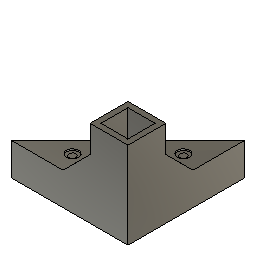
Rear Corner Bracket (Autodesk Fusion 360 design; units mm, degrees)
Autodesk Fusion 360 part; units mm, degrees
sketch "Sketch1" plane through (0, 0, 0) normal (0, 0, 1) x (1, 0, 0)
  line L0 (44, 14) -> (-44, 14)
  line L1 (-44, 14) -> (-44, -14)
  line L2 (-44, -14) -> (44, -14)
  line L3 (44, -14) -> (44, 14)
  line L4 (44, 14) -> (-44, -14) construction
  line L5 (-44, 14) -> (44, -14) construction
  dimension "d1" = 88
  dimension "d2" = 28
  constraint perpendicular L0 L1
  constraint parallel L0 L2
  constraint parallel L1 L3
  constraint horizontal L0
  constraint coincident L4 origin
  constraint coincident L5 origin
  measures "d1" distance of L1.end L2.end
  measures "d2" distance of L0.end L1.end
extrude "Extrude1" add sketch "Sketch1" along normal blind 24
sketch "Sketch2" plane through (0, 14, 0) normal (0, 1, 0) x (-1, 0, 0)
  line L0 (-44, 0) -> (44, 0)
  line L1 (44, 0) -> (44, 24)
  line L2 (44, 24) -> (-44, 24)
  line L3 (-44, 24) -> (-44, 0)
  line L4 (-44, 24) -> (-16, 24)
  line L5 (-16, 24) -> (-16, 0)
  line L6 (-16, 0) -> (-44, 0)
  line L7 (-44, 0) -> (-44, 24)
  dimension "d5" = 24
  dimension "d6" = 28
  constraint horizontal L4
  constraint vertical L5
  constraint horizontal L6
  constraint vertical L7
  constraint coincident L2.end L3.start
  measures "d5" distance of L2.end L0.start
  measures "d6" distance of L2.end L4.end
extrude "Extrude2" add sketch "Sketch2" along normal blind 60 contours L0 L2 L3 L4 L5 L6 L7
sketch "Sketch3" plane through (0, 0, 0) normal (0, 0, -1) x (1, 0, 0)
  line L0 (44, -74) -> (44, 14)
  line L1 (44, 14) -> (-44, 14)
  line L2 (-44, 14) -> (-44, -14)
  line L3 (-44, -14) -> (16, -14)
  line L4 (16, -14) -> (16, -74)
  line L5 (16, -74) -> (44, -74)
  line L6 (-44, 10) -> (44, 10) construction
  line L7 (-44, -10) -> (44, -10) construction
  line L8 (20, -74) -> (20, 14) construction
  line L9 (40, -74) -> (40, 14) construction
  line L10 (-44, 10) -> (40, 10)
  line L11 (40, 10) -> (40, -10)
  line L12 (40, -10) -> (-44, -10)
  line L13 (-44, -10) -> (-44, 10)
  line L14 (20, 10) -> (40, 10)
  line L15 (40, 10) -> (40, -74)
  line L16 (40, -74) -> (20, -74)
  line L17 (20, -74) -> (20, 10)
  dimension "d9" = 4
  dimension "d10" = 4
  dimension "d11" = 4
  dimension "d12" = 4
  constraint coincident L2 L6.start
  constraint coincident L0 L6.end
  constraint perpendicular L0 L6
  constraint coincident L2 L7.start
  constraint coincident L0 L7.end
  constraint perpendicular L0 L7
  constraint coincident L5 L8.start
  constraint coincident L1 L8.end
  constraint perpendicular L1 L8
  constraint coincident L5 L9.start
  constraint coincident L1 L9.end
  constraint perpendicular L1 L9
  constraint horizontal L10
  constraint vertical L11
  constraint horizontal L12
  constraint vertical L13
  constraint coincident L7 L11.end
  constraint coincident L9 L11.end
  constraint horizontal L14
  constraint vertical L15
  constraint horizontal L16
  constraint vertical L17
  constraint coincident L8 L14.start
  constraint coincident L10 L14.start
  measures "d9" distance of L0 L9
  measures "d10" distance of L4 L8
  measures "d11" distance of L3 L7
  measures "d12" distance of L1 L6
extrude "Extrude3" cut sketch "Sketch3" against normal blind 20 contours L5 L12 L15 L16 L17 | L10 L11 L12 L14 L15 L17 | L2 L10 L12 L13 L17
sketch "Sketch4" plane through (0, 0, 24) normal (0, 0, 1) x (-1, 0, 0)
  line L0 (-44, 14) -> (-44, -74)
  line L1 (-44, -74) -> (-16, -74)
  line L2 (-16, -74) -> (-16, -14)
  line L3 (-16, -14) -> (44, -14)
  line L4 (44, -14) -> (44, 14)
  line L5 (44, 14) -> (-44, 14)
  line L6 (14, -14) -> (-16, -44)
  constraint midpoint L3 L6.start
  constraint midpoint L2 L6.end
extrude "Extrude4" add sketch "Sketch4" against normal blind 4 contours L2 L3 L6
sketch "Sketch5" plane through (0, 0, 0) normal (0, 0, -1) x (1, 0, 0)
  line L0 (20, -10) -> (-44, -10)
  line L1 (-44, -10) -> (-44, -14)
  line L2 (-44, -14) -> (16, -14)
  line L3 (16, -14) -> (16, -74)
  line L4 (16, -74) -> (20, -74)
  line L5 (20, -74) -> (20, -10)
  line L6 (-14, -14) -> (16, -44)
  constraint midpoint L2 L6.start
  constraint midpoint L3 L6.end
extrude "Extrude5" add sketch "Sketch5" against normal blind 4 contours L2 L3 L6
sketch "Sketch6" plane through (0, 14, 0) normal (0, 1, 0) x (-1, 0, 0)
  line L0 (-16, 4) -> (14, 4)
  line L1 (14, 4) -> (14, 0)
  line L2 (14, 0) -> (44, 0)
  line L3 (44, 0) -> (44, 24)
  line L4 (44, 24) -> (14, 24)
  line L5 (14, 24) -> (14, 20)
  line L6 (14, 20) -> (-16, 20)
  line L7 (-16, 20) -> (-16, 4)
  line L8 (-6, 20) -> (-6, 4) construction
  line L9 (-16, 10) -> (44, 10) construction
  line L10 (14, 24) -> (-16, 24) construction
  circle A0 centre (-6, 10) radius 2.5
  circle A1 centre (-6, 10) radius 4.5
  dimension "d19" = 10
  dimension "d69" = 10
  dimension "d70" = 5
  dimension "d71" = 9
  constraint coincident L6 L8.start
  constraint coincident L0 L8.end
  constraint perpendicular L0 L8
  constraint coincident L7 L9.start
  constraint coincident L3 L9.end
  constraint perpendicular L3 L9
  constraint coincident L9 A0.centre
  constraint coincident L8 A0.centre
  constraint concentric A0 A1
  measures "d19" distance of L7 L8
  measures "d69" distance of L2 L9
  measures "d70" diameter of A0
  measures "d71" diameter of A1
extrude "Extrude36" cut sketch "Sketch6" against normal blind 1 contours A0 | A1
extrude "Extrude19" cut sketch "Sketch6" against normal blind 2.8 from surface at -1 contours A0
sketch "Sketch7" plane through (16, 0, 0) normal (-1, 0, 0) x (0, -1, 0)
  line L0 (-44, 0) -> (-44, 4)
  line L1 (-44, 4) -> (-14, 4)
  line L2 (-14, 4) -> (-14, 20)
  line L3 (-14, 20) -> (-44, 20)
  line L4 (-44, 20) -> (-44, 24)
  line L5 (-44, 24) -> (-74, 24)
  line L6 (-74, 24) -> (-74, 0)
  line L7 (-74, 0) -> (-44, 0)
  line L8 (-24, 20) -> (-24, 4) construction
  line L9 (-14, 20) -> (-14, 4) construction
  line L10 (-14, 10) -> (-74, 10) construction
  line L11 (-14, 24) -> (-44, 24) construction
  circle A0 centre (-24, 10) radius 2.5
  circle A1 centre (-24, 10) radius 4.5
  dimension "d26" = 10
  dimension "d62" = 5
  dimension "d63" = 9
  dimension "d76" = 10
  constraint coincident L3 L8.start
  constraint coincident L1 L8.end
  constraint perpendicular L1 L8
  constraint coincident L2 L10.start
  constraint coincident L6 L10.end
  constraint perpendicular L6 L10
  constraint coincident L8 A0.centre
  constraint coincident L10 A0.centre
  constraint concentric A0 A1
  measures "d26" distance of L8 L9
  measures "d62" diameter of A0
  measures "d63" diameter of A1
  measures "d76" distance of L7 L10
extrude "Extrude35" cut sketch "Sketch7" against normal blind 1 contours A0 | A1
extrude "Extrude17" cut sketch "Sketch7" against normal blind 2.8 from surface at -1 contours A0
sketch "Sketch8" plane through (0, 0, 24) normal (0, 0, 1) x (-1, 0, 0)
  line L0 (-44, 14) -> (-44, -74)
  line L1 (-44, -74) -> (-16, -74)
  line L2 (-16, -74) -> (-16, -44)
  line L3 (-16, -44) -> (14, -14)
  line L4 (14, -14) -> (44, -14)
  line L5 (44, -14) -> (44, 14)
  line L6 (44, 14) -> (-44, 14)
  line L7 (14, -14) -> (42, 14)
  line L8 (-16, -44) -> (-44, -72)
  constraint coincident L3.end L4.start
  constraint coincident L6 L7.end
  constraint parallel L3 L7
  constraint coincident L2.end L3.start
  constraint coincident L0 L8.end
  constraint parallel L3 L8
extrude "Extrude10" cut sketch "Sketch8" against normal blind 24 contours L0 L1 L2 L8 | L4 L5 L6 L7
sketch "Sketch11" plane through (0, 0, 24) normal (0, 0, 1) x (-1, 0, 0)
  line L0 (-44, -72) -> (42, 14)
  line L1 (42, 14) -> (-44, 14)
  line L2 (-44, 14) -> (-44, -72)
  line L3 (11, 14) -> (11, -17) construction
  line L4 (-44, -41) -> (-13, -41) construction
  line L5 (-30, 14) -> (-30, -58) construction
  line L6 (-44, 0) -> (28, 0) construction
  circle A0 centre (-30, -41) radius 2.5
  circle A1 centre (-30, -41) radius 4.5
  circle A2 centre (11, 0) radius 2.5
  circle A3 centre (11, 0) radius 4.5
  dimension "d49" = 55
  dimension "d50" = 55
  dimension "d51" = 14
  dimension "d52" = 14
  dimension "d53" = 5
  dimension "d54" = 9
  dimension "d55" = 5
  dimension "d56" = 9
  constraint coincident L1 L3.start
  constraint coincident L0 L3.end
  constraint perpendicular L1 L3
  constraint coincident L2 L4.start
  constraint coincident L0 L4.end
  constraint perpendicular L2 L4
  constraint coincident L1 L5.start
  constraint coincident L0 L5.end
  constraint perpendicular L1 L5
  constraint coincident L2 L6.start
  constraint coincident L0 L6.end
  constraint perpendicular L2 L6
  constraint coincident L4 A0.centre
  constraint coincident L5 A0.centre
  constraint concentric A0 A1
  constraint coincident L3 A2.centre
  constraint coincident L6 A2.centre
  constraint concentric A2 A3
  measures "d49" distance of L2 L3
  measures "d50" distance of L1 L4
  measures "d51" distance of L1 L6
  measures "d52" distance of L2 L5
  measures "d53" diameter of A0
  measures "d54" diameter of A1
  measures "d55" diameter of A2
  measures "d56" diameter of A3
extrude "Extrude16" cut sketch "Sketch11" against normal blind 1 contours A1 | A3
extrude "Extrude15" cut sketch "Sketch11" against normal blind 4 contours A0 | A2
sketch "Sketch13" plane through (0, 0, 23) normal (0, 0, 1) x (-1, 0, 0)
  circle A0 centre (-30, -41) radius 2.5
  circle A1 centre (-30, -41) radius 4.5
  circle A2 centre (-30, -41) radius 2.5
  circle A3 centre (-30, -41) radius 2.5
  constraint concentric A0 A2
  constraint concentric A2 A3
extrude "Extrude21" add sketch "Sketch11" against normal blind 0.2 from surface at -1 contours A0
sketch "Sketch14" plane through (0, 0, 23) normal (0, 0, 1) x (-1, 0, 0)
  circle A0 centre (11, 0) radius 2.5
  circle A1 centre (11, 0) radius 4.5
extrude "Extrude22" add sketch "Sketch11" along normal blind 0.2 from surface at -1.2 contours A2
sketch "Sketch16" plane through (0, 0, 24) normal (0, 0, 1) x (-1, 0, 0)
  circle A0 centre (11, 0) radius 4.5
  circle A1 centre (-30, -41) radius 4.5
  line L0 (-44, -72) -> (42, 14)
  line L1 (42, 14) -> (-44, 14)
  line L2 (-44, 14) -> (-44, -72)
  line L3 (-44, 14) -> (-16, 14)
  line L4 (-16, 14) -> (-16, -14)
  line L5 (-16, -14) -> (-44, -14)
  line L6 (-44, -14) -> (-44, 14)
  dimension "d83" = 28
  dimension "d84" = 28
  constraint horizontal L3
  constraint vertical L4
  constraint horizontal L5
  constraint vertical L6
  constraint coincident L1.end L2.start
  measures "d83" distance of L1.end L3.end
  measures "d84" distance of L1.end L5.end
extrude "Extrude23" add sketch "Sketch16" along normal blind 40 contours L1 L2 L3 L4 L5 L6
sketch "Sketch17" plane through (0, 0, 64) normal (0, 0, 1) x (-1, 0, 0)
  line L0 (-44, -14) -> (-16, -14)
  line L1 (-16, -14) -> (-16, 14)
  line L2 (-16, 14) -> (-44, 14)
  line L3 (-44, 14) -> (-44, -14)
  line L4 (-16, 0) -> (-18.5204, 0) construction
  line L5 (-18.5204, 0) -> (-44, 0) construction
  line L6 (-30, -14) -> (-30, 14) construction
  line L7 (-40, 10) -> (-20, 10)
  line L8 (-20, 10) -> (-20, -10)
  line L9 (-20, -10) -> (-40, -10)
  line L10 (-40, -10) -> (-40, 10)
  line L11 (-40, 10) -> (-20, -10) construction
  line L12 (-20, 10) -> (-40, -10) construction
  point P0 (-30, 0)
  dimension "d87" = 20
  dimension "d88" = 20
  constraint midpoint L1 L4.start
  constraint perpendicular L1 L4
  constraint midpoint L3 L5.end
  constraint perpendicular L3 L5
  constraint midpoint L0 L6.start
  constraint midpoint L2 L6.end
  constraint perpendicular L7 L8
  constraint parallel L7 L9
  constraint parallel L8 L10
  constraint horizontal L7
  constraint coincident L11 P0
  constraint coincident L12 P0
  constraint midpoint L6 P0
  measures "d87" distance of L8.end L9.end
  measures "d88" distance of L7.end L8.end
extrude "Extrude24" cut sketch "Sketch17" against normal blind 44 contours L7 L8 L9 L10
chamfer "Chamfer1" distance 20 angle 45 1 edges at (16, 0, 24)
chamfer "Chamfer2" distance 20 angle 45 1 edges at (20, 14, 24)
sketch "Sketch19" plane through (0, 0, 20) normal (0, 0, -1) x (1, 0, 0)
  circle A0 centre (-11, 0) radius 2.5
  line L0 (20, -10) -> (20, 10)
  line L1 (20, 10) -> (-38, 10)
  line L2 (-38, 10) -> (-18, -10)
  line L3 (-18, -10) -> (20, -10)
  line L4 (-4, 10) -> (-4, -10)
  line L5 (16, 10) -> (16, -10)
  line L6 (-4, 10) -> (16, 10)
  line L7 (16, 10) -> (16, -10)
  line L8 (16, -10) -> (-4, -10)
  line L9 (-4, -10) -> (-4, 10)
  dimension "d95" = 4
  dimension "d96" = 24
  constraint coincident L1 L4.start
  constraint coincident L3 L4.end
  constraint perpendicular L3 L4
  constraint coincident L1 L5.start
  constraint coincident L3 L5.end
  constraint perpendicular L3 L5
  constraint horizontal L6
  constraint vertical L7
  constraint horizontal L8
  constraint vertical L9
  measures "d95" distance of L0 L5
  measures "d96" distance of L0 L4
extrude "Extrude25" cut sketch "Sketch19" against normal blind 20 from surface at -4 contours L1 L3 L4 L5 L6 L7 L8 L9
sketch "Sketch20" plane through (0, 0, 20) normal (0, 0, -1) x (1, 0, 0)
  circle A0 centre (30, -41) radius 2.5
  line L0 (40, -10) -> (20, -10)
  line L1 (20, -10) -> (20, -48)
  line L2 (20, -48) -> (40, -68)
  line L3 (40, -68) -> (40, -10)
  line L4 (40, -14) -> (20, -14)
  line L5 (40, -34) -> (20, -34)
  dimension "d100" = 4
  dimension "d101" = 24
  constraint coincident L3 L4.start
  constraint coincident L1 L4.end
  constraint perpendicular L1 L4
  constraint coincident L3 L5.start
  constraint coincident L1 L5.end
  constraint perpendicular L1 L5
  measures "d100" distance of L0 L4
  measures "d101" distance of L0 L5
extrude "Extrude26" cut sketch "Sketch20" against normal blind 20 from surface at -4 contours L1 L3 L4 L5
sketch "Sketch22" plane through (16, 0, 0) normal (-1, 0, 0) x (0, -1, 0)
  line L0 (10, 44) -> (14, 44)
  line L1 (14, 44) -> (14, 64)
  line L2 (14, 64) -> (-14, 64)
  line L3 (-14, 64) -> (-14, 44)
  line L4 (-14, 44) -> (-10, 44)
  line L5 (-10, 44) -> (-10, 24)
  line L6 (-10, 24) -> (10, 24)
  line L7 (10, 24) -> (10, 44)
  line L8 (0, 64) -> (0, 24) construction
  line L9 (-14, 44) -> (14, 44) construction
  circle A0 centre (0, 44) radius 2.5
  circle A1 centre (0, 44) radius 4.5
  dimension "d105" = 5
  dimension "d106" = 9
  constraint midpoint L2 L8.start
  constraint midpoint L6 L8.end
  constraint coincident L3.end L4.start
  constraint coincident L0.end L1.start
  constraint midpoint L8 A0.centre
  constraint concentric A0 A1
  measures "d105" diameter of A0
  measures "d106" diameter of A1
extrude "Extrude33" cut sketch "Sketch22" against normal blind 1 contours A0 | A1
extrude "Extrude27" cut sketch "Sketch22" against normal blind 2.8 from surface at -1 contours A0
sketch "Sketch23" plane through (0, 14, 0) normal (0, 1, 0) x (-1, 0, 0)
  line L0 (-20, 44) -> (-16, 44)
  line L1 (-16, 44) -> (-16, 64)
  line L2 (-16, 64) -> (-44, 64)
  line L3 (-44, 64) -> (-44, 44)
  line L4 (-44, 44) -> (-40, 44)
  line L5 (-40, 44) -> (-40, 24)
  line L6 (-40, 24) -> (-20, 24)
  line L7 (-20, 24) -> (-20, 44)
  line L8 (-30, 64) -> (-30, 24) construction
  line L9 (-44, 44) -> (-16, 44) construction
  circle A0 centre (-30, 44) radius 2.5
  circle A1 centre (-30, 44) radius 4.5
  dimension "d111" = 5
  dimension "d112" = 9
  constraint midpoint L2 L8.start
  constraint midpoint L6 L8.end
  constraint coincident L3.end L4.start
  constraint coincident L0.end L1.start
  constraint midpoint L9 A0.centre
  constraint concentric A0 A1
  measures "d111" diameter of A0
  measures "d112" diameter of A1
extrude "Extrude34" cut sketch "Sketch23" against normal blind 1 contours A0 | A1
extrude "Extrude29" cut sketch "Sketch23" against normal blind 2.8 from surface at -1 contours A0
extrude "Extrude31" add 1 faces at (-11.643, 0.1378, 22.8) along direction (0, 0, -1) blind 0.2 from surface at 2.6
extrude "Extrude32" add 1 faces at (30.5928, 42.1373, 22.8) along direction (0, 0, -1) blind 0.2 from surface at 2.6
